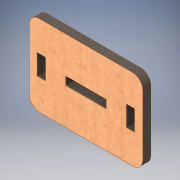
# Autodesk Inventor part: PistonPart5
Saved by Autodesk Inventor 2019 (Build 230136000, 136)
## iProperties
Created: 2021-01-03
Part Number: PistonPart5
Material: Дерево (вишня)
Document SubType Name: Modeling
Designer: Professional
Density: 0.63 g/cm^3
Appearance: Вишневое дерево — натуральный — со слабым глянцем
Author: Professional
Autodesk Inventor part; units mm, degrees
ref_plane "YZ Plane" through (0, 0, 0) normal (1, 0, 0) x (0, 1, 0)
ref_plane "XZ Plane" through (0, 0, 0) normal (0, 1, 0) x (-1, 0, 0)
ref_plane "XY Plane" through (0, 0, 0) normal (0, 0, 1) x (1, 0, 0)
sketch "Эскиз1" plane through (0, 0, 0) normal (0, 0, 1) x (1, 0, 0)
  line L0 (-25, 0) -> (25, 0) construction
  line L1 (-10, -2) -> (10, -2)
  line L2 (10, -2) -> (10, 2)
  line L3 (10, 2) -> (-10, 2)
  line L4 (-10, 2) -> (-10, -2)
  line L5 (-24, 5) -> (-20, 5)
  line L6 (-20, 5) -> (-20, -5)
  line L7 (-20, -5) -> (-24, -5)
  line L8 (-24, -5) -> (-24, 5)
  line L9 (0, 20) -> (0, -20) construction
  line L10 (24, 5) -> (20, 5)
  line L11 (20, 5) -> (20, -5)
  line L12 (20, -5) -> (24, -5)
  line L13 (24, -5) -> (24, 5)
  line L14 (-23, 20) -> (23, 20)
  line L15 (23, 20) -> (23, -20) construction
  line L16 (23, -20) -> (-23, -20)
  line L17 (-23, -20) -> (-23, 20) construction
  arc A0 (-23, 20) -> (-28, 15) centre (-23, 15) ccw
  arc A1 (-28, -15) -> (-23, -20) centre (-23, -15) ccw
  arc A2 (23, -20) -> (28, -15) centre (23, -15) ccw
  arc A3 (28, 15) -> (23, 20) centre (23, 15) ccw
  line L18 (-28, 15) -> (-28, -15)
  line L19 (28, -15) -> (28, 15)
  point P0 (0, 0)
  point P1 (-20, 0)
  point P2 (-10, 0)
  point P3 (0, -2)
  point P4 (0, 0)
  dimension "d0" = 4
  dimension "d1" = 40
  dimension "d2" = 20
  dimension "d3" = 10
  dimension "d4" = 50
  dimension "d6" = 56
  dimension "d7" = 40
  dimension "d8" = 5
  constraints: 42 end point, 8 point on circle, 7 midpoint, 7 parallel, 4 centre point, 4 horizontal, 4 perpendicular, 4 point on line, 4 symmetric about line, 3 equal radius, 2 horizontal alignment, 2 tangent, 1 coincident, 1 vertical, 1 vertical alignment, 1 other
  measures "d0" distance of L5.start L5.end
  measures "d1" distance between parallel lines of L11 L6
  measures "d2" distance between parallel lines of L2 L4
  measures "d3" distance between parallel lines of L12 L10
  measures "d4" distance of L0.end L0.start
  measures "d6" distance between parallel lines of L19 L18
  measures "d7" distance between parallel lines of L16 L14
  measures "d8" radius of A2
extrude "Выдавливание1" add sketch "Эскиз1" along normal blind 4
